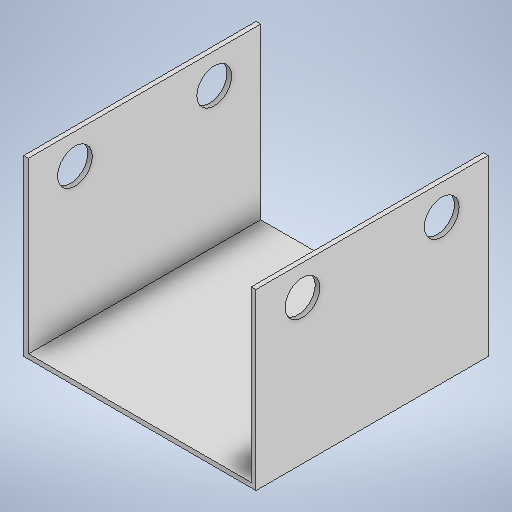
# Autodesk Inventor part: motor holder
Saved by Autodesk Inventor 2025.2 (Build 292293000, 293)
## iProperties
Created: 2025-02-17
Part Number: motor holder
Material: Generic
Document SubType Name: Modeling
Designer: Khushal
Density: 1 g/cm^3
Appearance: Default
Author: Khushal
Autodesk Inventor part; units mm, degrees
ref_plane "YZ Plane" through (0, 0, 0) normal (1, 0, 0) x (0, 1, 0)
ref_plane "XZ Plane" through (0, 0, 0) normal (0, 1, 0) x (-1, 0, 0)
ref_plane "XY Plane" through (0, 0, 0) normal (0, 0, 1) x (1, 0, 0)
sketch "Sketch1" plane through (0, 0, 0) normal (0, 0, 1) x (1, 0, 0)
  line L0 (0, 0) -> (0, 75)
  line L1 (0, 0) -> (100, 0)
  line L2 (100, 0) -> (100, 75)
  line L3 (0, 75) -> (2, 75)
  line L4 (2, 75) -> (2, 2)
  line L5 (2, 2) -> (98, 2)
  line L6 (98, 2) -> (98, 75)
  line L7 (98, 75) -> (100, 75)
  dimension "d0" = 75
  dimension "d1" = 100
  dimension "d2" = 75
  dimension "d3" = 2
  dimension "d4" = 73
  dimension "d5" = 96
  constraints: 16 end point, 2 horizontal, 2 parallel, 2 perpendicular, 1 point on line, 1 vertical
  measures "d0" distance of L0.start L0.end
  measures "d1" distance of L0.start L1.end
  measures "d2" distance of L1.end L2.end
  measures "d3" distance of L0.end L3.end
  measures "d4" distance of L3.end L4.end
  measures "d5" distance of L4.end L5.end
extrude "Extrusion1" add sketch "Sketch1" against normal blind 100
sketch "Sketch2" plane through (100, 0, 0) normal (1, 0, 0) x (0, 0, -1)
  line L0 (0, 75) -> (100, 75) projected
  line L1 (0, 75) -> (20, 75)
  line L2 (100, 2) -> (100, 75) projected
  line L3 (20, 75) -> (20, 62)
  line L4 (20, 62) -> (80, 62)
  circle A0 centre (20, 62) radius 7.5
  circle A1 centre (80, 62) radius 7.5
  point P0 (0, 0)
  dimension "d8" = 20
  dimension "d9" = 13
  dimension "d10" = 60
  dimension "d11" = 15
  dimension "d12" = 15
  constraints: 6 end point, 3 perpendicular, 2 centre point, 2 coincident
  measures "d8" distance of L0.start L1.end
  measures "d9" distance of L1.end L3.end
  measures "d10" distance of L3.end L4.end
  measures "d11" diameter of A0
  measures "d12" diameter of A1
extrude "Extrusion2" cut sketch "Sketch2" against normal through all
body "Solid1"
